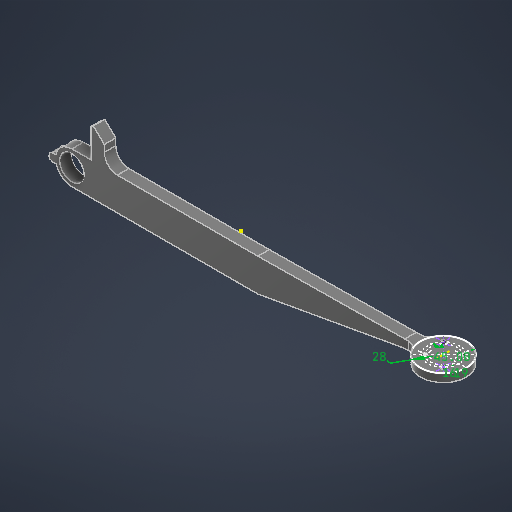
# Autodesk Inventor part: BOOM ARM
Saved by Autodesk Inventor 2025 (Build 290162010, 162A)
## iProperties
Created: 2025-05-21
Part Number: BOOM ARM
Material: Aluminum 6061
Document SubType Name: Modeling
Designer: Jebediah Kerman
Density: 2.7 g/cm^3
Appearance: Smooth - Black
Mass: 64.7238 g
Surface Area: 113.882 cm^2
Volume: 23.9718 cm^3
Author: Jebediah Kerman
Autodesk Inventor part; units mm, degrees
ref_plane "YZ Plane" through (0, 0, 0) normal (1, 0, 0) x (0, 1, 0)
ref_plane "XZ Plane" through (0, 0, 0) normal (0, 1, 0) x (-1, 0, 0)
ref_plane "XY Plane" through (0, 0, 0) normal (0, 0, 1) x (1, 0, 0)
sketch "Sketch1" plane through (0, 0, 0) normal (0, 0, 1) x (1, 0, 0)
  line L0 (107.2618, 7.9599) -> (127.2618, 7.9599)
  line L1 (127.2618, 7.9599) -> (127.2618, 2.9599)
  line L2 (127.2618, 2.9599) -> (107.2618, 2.9599)
  line L3 (107.2618, 2.9599) -> (107.2618, 7.9599)
  circle A0 centre (-95.9382, -3.1699) radius 7.5
  circle A1 centre (-95.9382, -3.1699) radius 10
  line L4 (-95.9382, -13.1699) -> (-67.2988, -13.1699)
  line L5 (-67.2988, -13.1699) -> (17.5278, -13.1699)
  line L6 (107.2618, 2.9599) -> (17.5278, -13.1699)
  line L7 (-95.9382, 6.8301) -> (17.5278, 6.8301)
  line L8 (17.5278, 6.8301) -> (107.2618, 7.9599)
  line L9 (-105.7312, -1.1457) -> (-107.876, -1.1457)
  line L10 (-109.876, -3.1457) -> (-109.876, -3.9908)
  line L11 (-107.876, -5.9908) -> (-105.5321, -5.9908)
  arc A2 (-107.876, -1.1457) -> (-109.876, -3.1457) centre (-107.876, -3.1457) ccw
  arc A3 (-109.876, -3.9908) -> (-107.876, -5.9908) centre (-107.876, -3.9908) ccw
  point P0 (0, 0)
  point P1 (107.2618, 5.4599)
  point P2 (-109.876, -5.9908)
  point P3 (-109.876, -1.1457)
  dimension "d0" = 20
  dimension "d1" = 15
  dimension "d2" = 203.2
  dimension "d3" = 20
  dimension "d4" = 5
  dimension "d43" = 2
  constraints: 24 end point, 8 point on circle, 6 tangent, 5 point on line, 4 centre point, 4 horizontal, 3 parallel, 2 perpendicular, 1 coincident, 1 equal radius, 1 midpoint
  measures "d0" distance of L1.end L2.end
  measures "d1" diameter of A0
  measures "d2" horizontal distance of point (107.262, 5.46) A0.centre
  measures "d3" diameter of A1
  measures "d4" distance of L0.end L1.end
  measures "d43" radius of A2
extrude "Extrusion1" add sketch "Sketch1" along normal blind 7
sketch "Sketch2" plane through (107.2618, 7.9599, 0) normal (0, 1, 0) x (1, 0, 0)
  line L0 (20, 0) -> (20, -7) projected
  circle A0 centre (20, -3.5) radius 14
  circle A1 centre (20, -3.5) radius 9.5 construction
  circle A2 centre (20, -3.5) radius 8 construction
  line L1 (20, -3.5) -> (29.8995, 6.3995) construction
  line L2 (20, -3.5) -> (34, -3.5) construction
  line L3 (20, -3.5) -> (10.1005, 6.3995) construction
  line L4 (20, -3.5) -> (10.1005, -13.3995) construction
  line L5 (20, -3.5) -> (29.8995, -13.3995) construction
  point P0 (-107.2618, 0)
  point P1 (13.2825, 3.2175)
  point P2 (26.7175, -10.2175)
  point P3 (25.6569, 2.1569)
  point P4 (14.3431, -9.1569)
  dimension "d7" = 28
  dimension "d8" = 19
  dimension "d9" = 16
  dimension "d10" = 45
  constraints: 10 end point, 8 point on circle, 6 point on line, 3 centre point, 2 coincident, 1 equal length, 1 horizontal, 1 midpoint
  measures "d7" diameter of A0
  measures "d8" diameter of A1
  measures "d9" diameter of A2
  measures "d10" angle of L2 L1
extrude "Extrusion2" add sketch "Sketch2" against normal blind 5
hole "Hole1" at (120.5443, 7.9599, -3.2175) at (133.9793, 7.9599, 10.2175) at (132.9187, 7.9599, -2.1569) at (121.605, 7.9599, 9.1569) direction (0, -1, 0) diameter 3 end through all
fillet "Fillet1" radius 6 2 edges at (113.7064, 5.4599, 7) (113.7064, 5.4599, 0)
sketch "Sketch4" plane through (0, 0, 7) normal (0, 0, 1) x (1, 0, 0)
  line L0 (17.5278, 6.8301) -> (-95.9382, 6.8301) projected
  line L1 (-76.1299, 6.8301) -> (-50.7299, 6.8301) construction
  line L2 (-76.1721, 18.9955) -> (-76.1721, 6.8301)
  line L3 (-76.1299, 6.8301) -> (-76.1721, 6.8301)
  line L4 (-76.1721, 6.8301) -> (-84.1721, 6.8301)
  line L5 (-84.1721, 6.8301) -> (-84.1721, 24.5167)
  line L6 (-76.1721, 18.9955) -> (-82.8508, 25.4621)
  line L7 (-82.8508, 25.4621) -> (-84.1721, 24.5167)
  point P0 (0, 0)
  dimension "d42" = 8
  constraints: 14 end point, 3 point on line, 2 perpendicular, 1 collinear, 1 horizontal
  measures "d42" distance of L2.end L4.end
extrude "Extrusion4" add sketch "Sketch4" against normal up to surface (7 mm away)
fillet "Fillet3" radius 8 1 edges at (-76.1721, 6.8301, 3.5)
body "Solid1"
